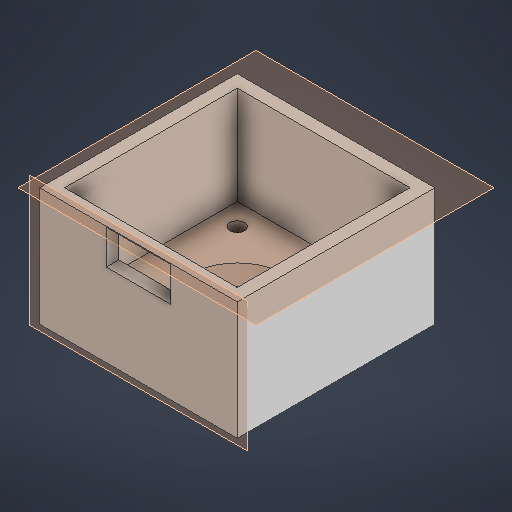
# Autodesk Inventor part: motor_case
Saved by Autodesk Inventor 2025.2 (Build 292293000, 293)
## iProperties
Created: 2024-11-24
Part Number: motor_case
Material: 一般
Document SubType Name: Modeling
Designer: dell
Density: 1 g/cm^3
Appearance: 既定
Author: dell
Autodesk Inventor part; units mm, degrees
ref_plane "YZ Plane" through (0, 0, 0) normal (1, 0, 0) x (0, 1, 0)
ref_plane "XZ Plane" through (0, 0, 0) normal (0, 1, 0) x (-1, 0, 0)
ref_plane "XY Plane" through (0, 0, 0) normal (0, 0, 1) x (1, 0, 0)
sketch "スケッチ1" plane through (0, 0, 0) normal (0, 1, 0) x (-1, 0, 0)
  line L0 (0, 0) -> (-47.5, 0)
  line L1 (-47.5, 0) -> (-47.5, -47.5)
  line L2 (-47.5, -47.5) -> (0, -47.5)
  line L3 (0, -47.5) -> (0, 0)
  dimension "d0" = 47.5
  dimension "d1" = 47.5
  constraints: 8 end point, 2 parallel, 1 horizontal, 1 perpendicular
  measures "d0" distance of L2.end L1.end
  measures "d1" distance of L1.end L0.end
extrude "押し出し1" add sketch "スケッチ1" along normal blind 28.4
ref_plane "作業平面1" through (0, 28.4, 0) normal (0, 1, 0) x (1, 0, 0)
sketch "スケッチ3" plane through (0, 28.4, 0) normal (0, 1, 0) x (1, 0, 0)
  line L0 (3, 3) -> (44.5, 3)
  line L1 (44.5, 3) -> (44.5, 44.5)
  line L2 (44.5, 44.5) -> (3, 44.5)
  line L3 (3, 44.5) -> (3, 3)
  line L4 (47.5, 47.5) -> (0, 47.5) projected
  line L5 (0, 47.5) -> (0, 0) projected
  dimension "d15" = 41.5
  dimension "d16" = 41.5
  dimension "d17" = 3
  dimension "d18" = 3
  constraints: 8 end point, 2 parallel, 1 horizontal, 1 perpendicular
  measures "d15" distance of L2.end L1.end
  measures "d16" distance of L1.end L0.end
  measures "d17" distance between parallel lines of L4 L2
  measures "d18" distance between parallel lines of L5 L3
extrude "押し出し3" cut sketch "スケッチ3" against normal blind 23.6
ref_plane "作業平面2" through (0, 4.8, 0) normal (0, 1, 0) x (1, 0, 0)
sketch "スケッチ4" plane through (0, 4.8, 0) normal (0, 1, 0) x (1, 0, 0)
  point P0 (0, 0)
  point P1 (23.75, 23.75)
hole "穴1" at (23.75, 4.8, -23.75) direction (0, -1, 0) diameter 22.5 end through all
sketch "スケッチ5" plane through (0, 4.8, 0) normal (0, 1, 0) x (1, 0, 0)
  line L0 (3, 44.5) -> (44.5, 44.5) projected
  line L1 (3, 3) -> (3, 44.5) projected
  line L2 (44.5, 44.5) -> (44.5, 3) projected
  line L3 (44.5, 3) -> (3, 3) projected
  point P0 (0, 0)
  point P1 (8.25, 39.25)
  point P2 (39.25, 39.25)
  point P3 (39.25, 8.25)
  point P4 (8.25, 8.25)
  dimension "d29" = 5.25
  dimension "d30" = 5.25
  dimension "d31" = 5.25
  dimension "d32" = 5.25
  dimension "d33" = 5.25
  dimension "d34" = 5.25
  dimension "d35" = 5.25
  dimension "d36" = 5.25
  measures "d29" distance from line of L0 point (8.25, 39.25)
  measures "d30" distance from line of L1 point (8.25, 39.25)
  measures "d31" distance from line of L2 point (39.25, 39.25)
  measures "d32" distance from line of L0 point (39.25, 39.25)
  measures "d33" distance from line of L2 point (39.25, 8.25)
  measures "d34" distance from line of L3 point (39.25, 8.25)
  measures "d35" distance from line of L3 point (8.25, 8.25)
  measures "d36" distance from line of L1 point (8.25, 8.25)
hole "穴2" at (8.25, 4.8, -39.25) at (39.25, 4.8, -39.25) at (39.25, 4.8, -8.25) at (8.25, 4.8, -8.25) direction (0, -1, 0) diameter 3.5 end through all
ref_plane "作業平面3" through (0, 0, 0) normal (0, 0, 1) x (1, 0, 0)
sketch "スケッチ6" plane through (0, 0, 0) normal (0, 0, 1) x (1, 0, 0)
  line L0 (16, 28.2) -> (31.5, 28.2)
  line L1 (31.5, 28.2) -> (31.5, 19.9)
  line L2 (31.5, 19.9) -> (16, 19.9)
  line L3 (16, 19.9) -> (16, 28.2)
  line L4 (0, 0) -> (47.5, 0) projected
  line L5 (0, 28.4) -> (47.5, 28.4) projected
  point P0 (23.75, 19.9)
  point P1 (23.75, 0)
  point P2 (23.75, 0)
  dimension "d46" = 19.9
  dimension "d47" = 0
  dimension "d48" = 15.5
  dimension "d51" = 8.5
  constraints: 8 end point, 3 midpoint, 2 parallel, 1 horizontal, 1 perpendicular, 1 other
  measures "d46" distance between parallel lines of L4 L2
  measures "d47" horizontal distance of point (23.75, 0) point (23.75, 19.9)
  measures "d48" distance of L1.end L2.end
extrude "押し出し4" cut sketch "スケッチ6" against normal blind 23.6
